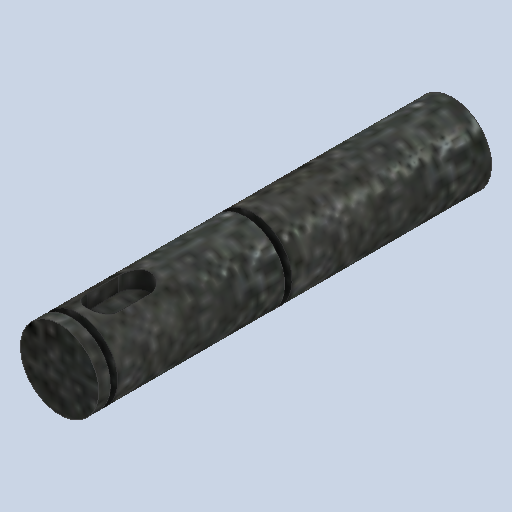
# Autodesk Inventor part: gearbox_shaft2
Saved by Autodesk Inventor 2023 (Build 270158000, 158)
## iProperties
Created: 2023-05-28
Part Number: gearbox_shaft2
Material: Steel
Document SubType Name: Modeling
Designer: 310611102
Density: 7.85 g/cm^3
Appearance: Plate
Mass: 29.7882 g
Surface Area: 19.0793 cm^2
Volume: 3.79468 cm^3
Vendor: 亞里士
Author: 310611102
Autodesk Inventor part; units mm, degrees
ref_plane "YZ Plane" through (0, 0, 0) normal (1, 0, 0) x (0, 1, 0)
ref_plane "XY Plane" through (0, 0, 0) normal (0, 0, 1) x (1, 0, 0)
sketch "Sketch5" plane through (0, 0, 0) normal (1, 0, 0) x (0, 1, 0)
  line L0 (0, 0) -> (5, 0)
  line L1 (5, 0) -> (5, -1.5)
  line L2 (5, -1.5) -> (3.55, -1.5)
  line L3 (3.55, -1.5) -> (3.55, -2.4)
  line L4 (3.55, -2.4) -> (5, -2.4)
  line L5 (5, -2.4) -> (5, -23.7)
  line L6 (5, -23.7) -> (3.55, -23.7)
  line L7 (3.55, -23.7) -> (3.55, -24.6)
  line L8 (3.55, -24.6) -> (5, -24.6)
  line L9 (5, -24.6) -> (5, -50)
  line L10 (5, -50) -> (0, -50)
  line L11 (0, -50) -> (0, 0)
  dimension "d14" = 0.9
  dimension "d15" = 1.5
  dimension "d16" = 0.9
  dimension "d17" = 50
  dimension "d18" = 10
  dimension "d19" = 7.1
  dimension "d28" = 23.1
  constraints: 24 end point, 9 perpendicular, 2 collinear, 2 horizontal, 2 point on line
  measures "d14" distance of L2.end L3.end
  measures "d15" distance of L0.end L1.end
  measures "d16" distance of L6.end L7.end
  measures "d17" distance between parallel lines of L0 L10
  measures "d18" diameter of L5 L11
  measures "d19" diameter of L7 L11
  measures "d28" distance between parallel lines of L2 L8
revolve "Revolution2" add sketch "Sketch5" angle 360 about axis through (0, 0, -50) along (0, 0, 1)
ref_plane "Work Plane1" through (0, 5, 0) normal (0, 1, 0) x (-1, 0, 0)
sketch "Sketch6" plane through (0, 5, 0) normal (0, 1, 0) x (-1, 0, 0)
  line L0 (0, -5.5) -> (0, -9.5) construction
  line L1 (-2, -5.5) -> (-2, -9.5)
  line L2 (2, -9.5) -> (2, -5.5)
  arc A0 (2, -5.5) -> (-2, -5.5) centre (0, -5.5) ccw
  arc A1 (-2, -9.5) -> (2, -9.5) centre (0, -9.5) ccw
  line L3 (5, -1.5) -> (-5, -1.5) projected
  point P0 (0, 0)
  point P1 (0, -7.5)
  point P2 (0, -3.5)
  point P3 (0, -11.5)
  dimension "d22" = 4
  dimension "d23" = 8
  dimension "d24" = 2
  constraints: 8 end point, 6 point on circle, 4 tangent, 2 centre point, 1 midpoint, 1 parallel, 1 vertical, 1 vertical alignment
  measures "d22" distance between parallel lines of L1 L2
  measures "d23" distance of point (0, -3.5) point (0, -11.5)
  measures "d24" distance from line of L3 point (0, -3.5)
extrude "Extrusion4" cut sketch "Sketch6" against normal blind 2.3
body "Solid2"
